Autodesk Fusion 360 part; units mm, degrees
(part 2 of 2)
  line L903 (-140.0079, -18.8092) -> (-138.8476, -19.992)
  line L904 (-137.1524, -16.008) -> (-138.8092, -15.9921)
  line L905 (-138.8092, -15.9921) -> (-139.992, -17.1524)
  line L906 (-139.992, -17.1524) -> (-140.0079, -18.8092)
  line L907 (-137.1908, -20.0079) -> (-136.008, -18.8476)
  line L908 (-146.8476, -19.992) -> (-145.1908, -20.0079)
  line L909 (-144.008, -18.8476) -> (-143.9921, -17.1908)
  line L910 (-143.9921, -17.1908) -> (-145.1524, -16.008)
  line L911 (-148.0079, -18.8092) -> (-146.8476, -19.992)
  line L912 (-145.1524, -16.008) -> (-146.8092, -15.9921)
  line L913 (-146.8092, -15.9921) -> (-147.992, -17.1524)
  line L914 (-147.992, -17.1524) -> (-148.0079, -18.8092)
  line L915 (-145.1908, -20.0079) -> (-144.008, -18.8476)
  line L916 (-154.8476, -19.992) -> (-153.1908, -20.0079)
  line L917 (-152.008, -18.8476) -> (-151.9921, -17.1908)
  line L918 (-151.9921, -17.1908) -> (-153.1524, -16.008)
  line L919 (-156.0079, -18.8092) -> (-154.8476, -19.992)
  line L920 (-153.1524, -16.008) -> (-154.8092, -15.9921)
  line L921 (-154.8092, -15.9921) -> (-155.992, -17.1524)
  line L922 (-155.992, -17.1524) -> (-156.0079, -18.8092)
  line L923 (-153.1908, -20.0079) -> (-152.008, -18.8476)
  line L924 (-162.8476, -19.992) -> (-161.1908, -20.0079)
  line L925 (-160.008, -18.8476) -> (-159.9921, -17.1908)
  line L926 (-159.9921, -17.1908) -> (-161.1524, -16.008)
  line L927 (-164.0079, -18.8092) -> (-162.8476, -19.992)
  line L928 (-161.1524, -16.008) -> (-162.8092, -15.9921)
  line L929 (-162.8092, -15.9921) -> (-163.992, -17.1524)
  line L930 (-163.992, -17.1524) -> (-164.0079, -18.8092)
  line L931 (-161.1908, -20.0079) -> (-160.008, -18.8476)
  line L932 (-170.8476, -19.992) -> (-169.1908, -20.0079)
  line L933 (-168.008, -18.8476) -> (-167.9921, -17.1908)
  line L934 (-167.9921, -17.1908) -> (-169.1524, -16.008)
  line L935 (-172.0079, -18.8092) -> (-170.8476, -19.992)
  line L936 (-169.1524, -16.008) -> (-170.8092, -15.9921)
  line L937 (-170.8092, -15.9921) -> (-171.992, -17.1524)
  line L938 (-171.992, -17.1524) -> (-172.0079, -18.8092)
  line L939 (-169.1908, -20.0079) -> (-168.008, -18.8476)
  line L940 (-10.8476, -11.992) -> (-9.1908, -12.0079)
  line L941 (-8.008, -10.8476) -> (-7.9921, -9.1908)
  line L942 (-7.9921, -9.1908) -> (-9.1524, -8.008)
  line L943 (-12.0079, -10.8092) -> (-10.8476, -11.992)
  line L944 (-9.1524, -8.008) -> (-10.8092, -7.9921)
  line L945 (-10.8092, -7.9921) -> (-11.992, -9.1524)
  line L946 (-11.992, -9.1524) -> (-12.0079, -10.8092)
  line L947 (-9.1908, -12.0079) -> (-8.008, -10.8476)
  line L948 (-18.8476, -11.992) -> (-17.1908, -12.0079)
  line L949 (-16.008, -10.8476) -> (-15.9921, -9.1908)
  line L950 (-15.9921, -9.1908) -> (-17.1524, -8.008)
  line L951 (-20.0079, -10.8092) -> (-18.8476, -11.992)
  line L952 (-17.1524, -8.008) -> (-18.8092, -7.9921)
  line L953 (-18.8092, -7.9921) -> (-19.992, -9.1524)
  line L954 (-19.992, -9.1524) -> (-20.0079, -10.8092)
  line L955 (-17.1908, -12.0079) -> (-16.008, -10.8476)
  line L956 (-26.8476, -11.992) -> (-25.1908, -12.0079)
  line L957 (-24.008, -10.8476) -> (-23.9921, -9.1908)
  line L958 (-23.9921, -9.1908) -> (-25.1524, -8.008)
  line L959 (-28.0079, -10.8092) -> (-26.8476, -11.992)
  line L960 (-25.1524, -8.008) -> (-26.8092, -7.9921)
  line L961 (-26.8092, -7.9921) -> (-27.992, -9.1524)
  line L962 (-27.992, -9.1524) -> (-28.0079, -10.8092)
  line L963 (-25.1908, -12.0079) -> (-24.008, -10.8476)
  line L964 (-34.8476, -11.992) -> (-33.1908, -12.0079)
  line L965 (-32.008, -10.8476) -> (-31.9921, -9.1908)
  line L966 (-31.9921, -9.1908) -> (-33.1524, -8.008)
  line L967 (-36.0079, -10.8092) -> (-34.8476, -11.992)
  line L968 (-33.1524, -8.008) -> (-34.8092, -7.9921)
  line L969 (-34.8092, -7.9921) -> (-35.992, -9.1524)
  line L970 (-35.992, -9.1524) -> (-36.0079, -10.8092)
  line L971 (-33.1908, -12.0079) -> (-32.008, -10.8476)
  line L972 (-42.8476, -11.992) -> (-41.1908, -12.0079)
  line L973 (-40.008, -10.8476) -> (-39.9921, -9.1908)
  line L974 (-39.9921, -9.1908) -> (-41.1524, -8.008)
  line L975 (-44.0079, -10.8092) -> (-42.8476, -11.992)
  line L976 (-41.1524, -8.008) -> (-42.8092, -7.9921)
  line L977 (-42.8092, -7.9921) -> (-43.992, -9.1524)
  line L978 (-43.992, -9.1524) -> (-44.0079, -10.8092)
  line L979 (-41.1908, -12.0079) -> (-40.008, -10.8476)
  line L980 (-50.8476, -11.992) -> (-49.1908, -12.0079)
  line L981 (-48.008, -10.8476) -> (-47.9921, -9.1908)
  line L982 (-47.9921, -9.1908) -> (-49.1524, -8.008)
  line L983 (-52.0079, -10.8092) -> (-50.8476, -11.992)
  line L984 (-49.1524, -8.008) -> (-50.8092, -7.9921)
  line L985 (-50.8092, -7.9921) -> (-51.992, -9.1524)
  line L986 (-51.992, -9.1524) -> (-52.0079, -10.8092)
  line L987 (-49.1908, -12.0079) -> (-48.008, -10.8476)
  line L988 (-58.8476, -11.992) -> (-57.1908, -12.0079)
  line L989 (-56.008, -10.8476) -> (-55.9921, -9.1908)
  line L990 (-55.9921, -9.1908) -> (-57.1524, -8.008)
  line L991 (-60.0079, -10.8092) -> (-58.8476, -11.992)
  line L992 (-57.1524, -8.008) -> (-58.8092, -7.9921)
  line L993 (-58.8092, -7.9921) -> (-59.992, -9.1524)
  line L994 (-59.992, -9.1524) -> (-60.0079, -10.8092)
  line L995 (-57.1908, -12.0079) -> (-56.008, -10.8476)
  line L996 (-66.8476, -11.992) -> (-65.1908, -12.0079)
  line L997 (-64.008, -10.8476) -> (-63.9921, -9.1908)
  line L998 (-63.9921, -9.1908) -> (-65.1524, -8.008)
  line L999 (-68.0079, -10.8092) -> (-66.8476, -11.992)
  line L1000 (-65.1524, -8.008) -> (-66.8092, -7.9921)
  line L1001 (-66.8092, -7.9921) -> (-67.992, -9.1524)
  line L1002 (-67.992, -9.1524) -> (-68.0079, -10.8092)
  line L1003 (-65.1908, -12.0079) -> (-64.008, -10.8476)
  line L1004 (-74.8476, -11.992) -> (-73.1908, -12.0079)
  line L1005 (-72.008, -10.8476) -> (-71.9921, -9.1908)
  line L1006 (-71.9921, -9.1908) -> (-73.1524, -8.008)
  line L1007 (-76.0079, -10.8092) -> (-74.8476, -11.992)
  line L1008 (-73.1524, -8.008) -> (-74.8092, -7.9921)
  line L1009 (-74.8092, -7.9921) -> (-75.992, -9.1524)
  line L1010 (-75.992, -9.1524) -> (-76.0079, -10.8092)
  line L1011 (-73.1908, -12.0079) -> (-72.008, -10.8476)
  line L1012 (-82.8476, -11.992) -> (-81.1908, -12.0079)
  line L1013 (-80.008, -10.8476) -> (-79.9921, -9.1908)
  line L1014 (-79.9921, -9.1908) -> (-81.1524, -8.008)
  line L1015 (-84.0079, -10.8092) -> (-82.8476, -11.992)
  line L1016 (-81.1524, -8.008) -> (-82.8092, -7.9921)
  line L1017 (-82.8092, -7.9921) -> (-83.992, -9.1524)
  line L1018 (-83.992, -9.1524) -> (-84.0079, -10.8092)
  line L1019 (-81.1908, -12.0079) -> (-80.008, -10.8476)
  line L1020 (-90.8476, -11.992) -> (-89.1908, -12.0079)
  line L1021 (-88.008, -10.8476) -> (-87.9921, -9.1908)
  line L1022 (-87.9921, -9.1908) -> (-89.1524, -8.008)
  line L1023 (-92.0079, -10.8092) -> (-90.8476, -11.992)
  line L1024 (-89.1524, -8.008) -> (-90.8092, -7.9921)
  line L1025 (-90.8092, -7.9921) -> (-91.992, -9.1524)
  line L1026 (-91.992, -9.1524) -> (-92.0079, -10.8092)
  line L1027 (-89.1908, -12.0079) -> (-88.008, -10.8476)
  line L1028 (-98.8476, -11.992) -> (-97.1908, -12.0079)
  line L1029 (-96.008, -10.8476) -> (-95.9921, -9.1908)
  line L1030 (-95.9921, -9.1908) -> (-97.1524, -8.008)
  line L1031 (-100.0079, -10.8092) -> (-98.8476, -11.992)
  line L1032 (-97.1524, -8.008) -> (-98.8092, -7.9921)
  line L1033 (-98.8092, -7.9921) -> (-99.992, -9.1524)
  line L1034 (-99.992, -9.1524) -> (-100.0079, -10.8092)
  line L1035 (-97.1908, -12.0079) -> (-96.008, -10.8476)
  line L1036 (-106.8476, -11.992) -> (-105.1908, -12.0079)
  line L1037 (-104.008, -10.8476) -> (-103.9921, -9.1908)
  line L1038 (-103.9921, -9.1908) -> (-105.1524, -8.008)
  line L1039 (-108.0079, -10.8092) -> (-106.8476, -11.992)
  line L1040 (-105.1524, -8.008) -> (-106.8092, -7.9921)
  line L1041 (-106.8092, -7.9921) -> (-107.992, -9.1524)
  line L1042 (-107.992, -9.1524) -> (-108.0079, -10.8092)
  line L1043 (-105.1908, -12.0079) -> (-104.008, -10.8476)
  line L1044 (-114.8476, -11.992) -> (-113.1908, -12.0079)
  line L1045 (-112.008, -10.8476) -> (-111.9921, -9.1908)
  line L1046 (-111.9921, -9.1908) -> (-113.1524, -8.008)
  line L1047 (-116.0079, -10.8092) -> (-114.8476, -11.992)
  line L1048 (-113.1524, -8.008) -> (-114.8092, -7.9921)
  line L1049 (-114.8092, -7.9921) -> (-115.992, -9.1524)
  line L1050 (-115.992, -9.1524) -> (-116.0079, -10.8092)
  line L1051 (-113.1908, -12.0079) -> (-112.008, -10.8476)
  line L1052 (-122.8476, -11.992) -> (-121.1908, -12.0079)
  line L1053 (-120.008, -10.8476) -> (-119.9921, -9.1908)
  line L1054 (-119.9921, -9.1908) -> (-121.1524, -8.008)
  line L1055 (-124.0079, -10.8092) -> (-122.8476, -11.992)
  line L1056 (-121.1524, -8.008) -> (-122.8092, -7.9921)
  line L1057 (-122.8092, -7.9921) -> (-123.992, -9.1524)
  line L1058 (-123.992, -9.1524) -> (-124.0079, -10.8092)
  line L1059 (-121.1908, -12.0079) -> (-120.008, -10.8476)
  line L1060 (-130.8476, -11.992) -> (-129.1908, -12.0079)
  line L1061 (-128.008, -10.8476) -> (-127.9921, -9.1908)
  line L1062 (-127.9921, -9.1908) -> (-129.1524, -8.008)
  line L1063 (-132.0079, -10.8092) -> (-130.8476, -11.992)
  line L1064 (-129.1524, -8.008) -> (-130.8092, -7.9921)
  line L1065 (-130.8092, -7.9921) -> (-131.992, -9.1524)
  line L1066 (-131.992, -9.1524) -> (-132.0079, -10.8092)
  line L1067 (-129.1908, -12.0079) -> (-128.008, -10.8476)
  line L1068 (-138.8476, -11.992) -> (-137.1908, -12.0079)
  line L1069 (-136.008, -10.8476) -> (-135.9921, -9.1908)
  line L1070 (-135.9921, -9.1908) -> (-137.1524, -8.008)
  line L1071 (-140.0079, -10.8092) -> (-138.8476, -11.992)
  line L1072 (-137.1524, -8.008) -> (-138.8092, -7.9921)
  line L1073 (-138.8092, -7.9921) -> (-139.992, -9.1524)
  line L1074 (-139.992, -9.1524) -> (-140.0079, -10.8092)
  line L1075 (-137.1908, -12.0079) -> (-136.008, -10.8476)
  line L1076 (-146.8476, -11.992) -> (-145.1908, -12.0079)
  line L1077 (-144.008, -10.8476) -> (-143.9921, -9.1908)
  line L1078 (-143.9921, -9.1908) -> (-145.1524, -8.008)
  line L1079 (-148.0079, -10.8092) -> (-146.8476, -11.992)
  line L1080 (-145.1524, -8.008) -> (-146.8092, -7.9921)
  line L1081 (-146.8092, -7.9921) -> (-147.992, -9.1524)
  line L1082 (-147.992, -9.1524) -> (-148.0079, -10.8092)
  line L1083 (-145.1908, -12.0079) -> (-144.008, -10.8476)
  line L1084 (-154.8476, -11.992) -> (-153.1908, -12.0079)
  line L1085 (-152.008, -10.8476) -> (-151.9921, -9.1908)
  line L1086 (-151.9921, -9.1908) -> (-153.1524, -8.008)
  line L1087 (-156.0079, -10.8092) -> (-154.8476, -11.992)
  line L1088 (-153.1524, -8.008) -> (-154.8092, -7.9921)
  line L1089 (-154.8092, -7.9921) -> (-155.992, -9.1524)
  line L1090 (-155.992, -9.1524) -> (-156.0079, -10.8092)
  line L1091 (-153.1908, -12.0079) -> (-152.008, -10.8476)
  line L1092 (-162.8476, -11.992) -> (-161.1908, -12.0079)
  line L1093 (-160.008, -10.8476) -> (-159.9921, -9.1908)
  line L1094 (-159.9921, -9.1908) -> (-161.1524, -8.008)
  line L1095 (-164.0079, -10.8092) -> (-162.8476, -11.992)
  line L1096 (-161.1524, -8.008) -> (-162.8092, -7.9921)
  line L1097 (-162.8092, -7.9921) -> (-163.992, -9.1524)
  line L1098 (-163.992, -9.1524) -> (-164.0079, -10.8092)
  line L1099 (-161.1908, -12.0079) -> (-160.008, -10.8476)
  line L1100 (-170.8476, -11.992) -> (-169.1908, -12.0079)
  line L1101 (-168.008, -10.8476) -> (-167.9921, -9.1908)
  line L1102 (-167.9921, -9.1908) -> (-169.1524, -8.008)
  line L1103 (-172.0079, -10.8092) -> (-170.8476, -11.992)
  line L1104 (-169.1524, -8.008) -> (-170.8092, -7.9921)
  line L1105 (-170.8092, -7.9921) -> (-171.992, -9.1524)
  line L1106 (-171.992, -9.1524) -> (-172.0079, -10.8092)
  line L1107 (-169.1908, -12.0079) -> (-168.008, -10.8476)
  point P0 (-10, -50)
  point P1 (-18, -50)
  point P2 (-26, -50)
  point P3 (-34, -50)
  point P4 (-42, -50)
  point P5 (-50, -50)
  point P6 (-58, -50)
  point P7 (-66, -50)
  point P8 (-74, -50)
  point P9 (-82, -50)
  point P10 (-90, -50)
  point P11 (-98, -50)
  point P12 (-106, -50)
  point P13 (-114, -50)
  point P14 (-122, -50)
  point P15 (-130, -50)
  point P16 (-138, -50)
  point P17 (-146, -50)
  point P18 (-154, -50)
  point P19 (-162, -50)
  point P20 (-170, -50)
  point P21 (-10, -42)
  point P22 (-18, -42)
  point P23 (-26, -42)
  point P24 (-34, -42)
  point P25 (-42, -42)
  point P26 (-50, -42)
  point P27 (-58, -42)
  point P28 (-66, -42)
  point P29 (-74, -42)
  point P30 (-82, -42)
  point P31 (-90, -42)
  point P32 (-98, -42)
  point P33 (-106, -42)
  point P34 (-114, -42)
  point P35 (-122, -42)
  point P36 (-130, -42)
  point P37 (-138, -42)
  point P38 (-146, -42)
  point P39 (-154, -42)
  point P40 (-162, -42)
  point P41 (-170, -42)
  point P42 (-10, -34)
  point P43 (-18, -34)
  point P44 (-26, -34)
  point P45 (-34, -34)
  point P46 (-42, -34)
  point P47 (-50, -34)
  point P48 (-58, -34)
  point P49 (-66, -34)
  point P50 (-74, -34)
  point P51 (-82, -34)
  point P52 (-90, -34)
  point P53 (-98, -34)
  point P54 (-106, -34)
  point P55 (-114, -34)
  point P56 (-122, -34)
  point P57 (-130, -34)
  point P58 (-138, -34)
  point P59 (-146, -34)
  point P60 (-154, -34)
  point P61 (-162, -34)
  point P62 (-170, -34)
  point P63 (-10, -26)
  point P64 (-18, -26)
  point P65 (-26, -26)
  point P66 (-34, -26)
  point P67 (-42, -26)
  point P68 (-50, -26)
  point P69 (-58, -26)
  point P70 (-66, -26)
  point P71 (-74, -26)
  point P72 (-82, -26)
  point P73 (-90, -26)
  point P74 (-98, -26)
  point P75 (-106, -26)
  point P76 (-114, -26)
  point P77 (-122, -26)
  point P78 (-130, -26)
  point P79 (-138, -26)
  point P80 (-146, -26)
  point P81 (-154, -26)
  point P82 (-162, -26)
  point P83 (-170, -26)
  point P84 (-10, -18)
  point P85 (-18, -18)
  point P86 (-26, -18)
  point P87 (-34, -18)
  point P88 (-42, -18)
  point P89 (-50, -18)
  point P90 (-58, -18)
  point P91 (-66, -18)
  point P92 (-74, -18)
  point P93 (-82, -18)
  point P94 (-90, -18)
  point P95 (-98, -18)
  point P96 (-106, -18)
  point P97 (-114, -18)
  point P98 (-122, -18)
  point P99 (-130, -18)
  point P100 (-138, -18)
  point P101 (-146, -18)
  point P102 (-154, -18)
  point P103 (-162, -18)
  point P104 (-170, -18)
  point P105 (-10, -10)
  point P106 (-18, -10)
  point P107 (-26, -10)
  point P108 (-34, -10)
  point P109 (-42, -10)
  point P110 (-50, -10)
  point P111 (-58, -10)
  point P112 (-66, -10)
  point P113 (-74, -10)
  point P114 (-82, -10)
  point P115 (-90, -10)
  point P116 (-98, -10)
  point P117 (-106, -10)
  point P118 (-114, -10)
  point P119 (-122, -10)
  point P120 (-130, -10)
  point P121 (-138, -10)
  point P122 (-146, -10)
  point P123 (-154, -10)
  point P124 (-162, -10)
  point P125 (-170, -10)
  dimension "d5" = 5
  dimension "d6" = 2
  dimension "d9" = -20
  dimension "d10" = -54
  dimension "d11" = 5
  dimension "d12" = 2
  dimension "d13" = 2
  dimension "d14" = 2
  dimension "d15" = 10
  dimension "d18" = -174
  dimension "d19" = -20
  dimension "d39" = 2
  dimension "d40" = 10
  dimension "d41" = 10
  dimension "d44" = -8
  dimension "d45" = 8
  constraint horizontal L4
  constraint vertical L5
  constraint horizontal L6
  constraint vertical L7
  constraint horizontal L76
  constraint vertical L77
  constraint horizontal L78
  constraint vertical L79
  measures "d5" distance of L0 L7
  measures "d6" distance of L1 L4
  measures "d11" distance of L1 L76
  measures "d12" distance of L0 L79
  measures "d13" distance of L76.start L76.end
  measures "d14" distance of L4.start L6.end
  measures "d15" distance of L76.start L78.end
  measures "d39" distance of P0 L107
  measures "d40" distance of L3 P0
  measures "d41" distance of L0 P0
extrude "Extrude2" cut sketch "Sketch2" against normal blind 5 contours L4 L5 L6 L7 | L8 L9 L10 L11 | L12 L13 L14 L15 | L16 L17 L18 L19 | L20 L21 L22 L23 | L24 L25 L26 L27 | L28 L29 L30 L31 | L32 L33 L34 L35 | L36 L37 L38 L39 | L40 L41 L42 L43 | L44 L45 L46 L47 | L48 L49 L50 L51 | L52 L53 L54 L55 | L56 L57 L58 L59 | L60 L61 L62 L63 | L64 L65 L66 L67 | L68 L69 L70 L71 | L72 L73 L74 L75 | L76 L77 L78 L79 | L80 L81 L82 L83 | L84 L85 L86 L87 | L88 L89 L90 L91 | L92 L93 L94 L95 | L96 L97 L98 L99 | L100 L101 L102 L103 L104 L105 L106 L107 | L108 L109 L110 L111 L112 L113 L114 L115 | L116 L117 L118 L119 L120 L121 L122 L123 | L124 L125 L126 L127 L128 L129 L130 L131 | L132 L133 L134 L135 L136 L137 L138 L139 | L140 L141 L142 L143 L144 L145 L146 L147 | L148 L149 L150 L151 L152 L153 L154 L155 | L156 L157 L158 L159 L160 L161 L162 L163 | L164 L165 L166 L167 L168 L169 L170 L171 | L172 L173 L174 L175 L176 L177 L178 L179 | L180 L181 L182 L183 L184 L185 L186 L187 | L188 L189 L190 L191 L192 L193 L194 L195 | L196 L197 L198 L199 L200 L201 L202 L203 | L204 L205 L206 L207 L208 L209 L210 L211 | L212 L213 L214 L215 L216 L217 L218 L219 | L220 L221 L222 L223 L224 L225 L226 L227 | L228 L229 L230 L231 L232 L233 L234 L235 | L236 L237 L238 L239 L240 L241 L242 L243 | L244 L245 L246 L247 L248 L249 L250 L251 | L252 L253 L254 L255 L256 L257 L258 L259 | L260 L261 L262 L263 L264 L265 L266 L267 | L268 L269 L270 L271 L272 L273 L274 L275 | L276 L277 L278 L279 L280 L281 L282 L283 | L284 L285 L286 L287 L288 L289 L290 L291 | L292 L293 L294 L295 L296 L297 L298 L299 | L300 L301 L302 L303 L304 L305 L306 L307 | L308 L309 L310 L311 L312 L313 L314 L315 | L316 L317 L318 L319 L320 L321 L322 L323 | L324 L325 L326 L327 L328 L329 L330 L331 | L332 L333 L334 L335 L336 L337 L338 L339 | L340 L341 L342 L343 L344 L345 L346 L347 | L348 L349 L350 L351 L352 L353 L354 L355 | L356 L357 L358 L359 L360 L361 L362 L363 | L364 L365 L366 L367 L368 L369 L370 L371 | L372 L373 L374 L375 L376 L377 L378 L379 | L380 L381 L382 L383 L384 L385 L386 L387 | L388 L389 L390 L391 L392 L393 L394 L395 | L396 L397 L398 L399 L400 L401 L402 L403 | L404 L405 L406 L407 L408 L409 L410 L411 | L412 L413 L414 L415 L416 L417 L418 L419 | L420 L421 L422 L423 L424 L425 L426 L427 | L428 L429 L430 L431 L432 L433 L434 L435 | L436 L437 L438 L439 L440 L441 L442 L443 | L444 L445 L446 L447 L448 L449 L450 L451 | L452 L453 L454 L455 L456 L457 L458 L459 | L460 L461 L462 L463 L464 L465 L466 L467 | L468 L469 L470 L471 L472 L473 L474 L475 | L476 L477 L478 L479 L480 L481 L482 L483 | L484 L485 L486 L487 L488 L489 L490 L491 | L492 L493 L494 L495 L496 L497 L498 L499 | L500 L501 L502 L503 L504 L505 L506 L507 | L508 L509 L510 L511 L512 L513 L514 L515 | L516 L517 L518 L519 L520 L521 L522 L523 | L524 L525 L526 L527 L528 L529 L530 L531 | L532 L533 L534 L535 L536 L537 L538 L539 | L540 L541 L542 L543 L544 L545 L546 L547 | L548 L549 L550 L551 L552 L553 L554 L555 | L556 L557 L558 L559 L560 L561 L562 L563 | L564 L565 L566 L567 L568 L569 L570 L571 | L572 L573 L574 L575 L576 L577 L578 L579 | L580 L581 L582 L583 L584 L585 L586 L587 | L588 L589 L590 L591 L592 L593 L594 L595 | L596 L597 L598 L599 L600 L601 L602 L603 | L604 L605 L606 L607 L608 L609 L610 L611 | L612 L613 L614 L615 L616 L617 L618 L619 | L620 L621 L622 L623 L624 L625 L626 L627 | L628 L629 L630 L631 L632 L633 L634 L635 | L636 L637 L638 L639 L640 L641 L642 L643 | L644 L645 L646 L647 L648 L649 L650 L651 | L652 L653 L654 L655 L656 L657 L658 L659 | L660 L661 L662 L663 L664 L665 L666 L667 | L668 L669 L670 L671 L672 L673 L674 L675 | L676 L677 L678 L679 L680 L681 L682 L683 | L684 L685 L686 L687 L688 L689 L690 L691 | L692 L693 L694 L695 L696 L697 L698 L699 | L700 L701 L702 L703 L704 L705 L706 L707 | L708 L709 L710 L711 L712 L713 L714 L715 | L716 L717 L718 L719 L720 L721 L722 L723 | L724 L725 L726 L727 L728 L729 L730 L731 | L732 L733 L734 L735 L736 L737 L738 L739 | L740 L741 L742 L743 L744 L745 L746 L747 | L748 L749 L750 L751 L752 L753 L754 L755 | L756 L757 L758 L759 L760 L761 L762 L763 | L764 L765 L766 L767 L768 L769 L770 L771 | L772 L773 L774 L775 L776 L777 L778 L779 | L780 L781 L782 L783 L784 L785 L786 L787 | L788 L789 L790 L791 L792 L793 L794 L795 | L796 L797 L798 L799 L800 L801 L802 L803 | L804 L805 L806 L807 L808 L809 L810 L811 | L812 L813 L814 L815 L816 L817 L818 L819 | L820 L821 L822 L823 L824 L825 L826 L827 | L828 L829 L830 L831 L832 L833 L834 L835 | L836 L837 L838 L839 L840 L841 L842 L843 | L844 L845 L846 L847 L848 L849 L850 L851 | L852 L853 L854 L855 L856 L857 L858 L859 | L860 L861 L862 L863 L864 L865 L866 L867 | L868 L869 L870 L871 L872 L873 L874 L875 | L876 L877 L878 L879 L880 L881 L882 L883 | L884 L885 L886 L887 L888 L889 L890 L891 | L892 L893 L894 L895 L896 L897 L898 L899 | L900 L901 L902 L903 L904 L905 L906 L907 | L908 L909 L910 L911 L912 L913 L914 L915 | L916 L917 L918 L919 L920 L921 L922 L923 | L924 L925 L926 L927 L928 L929 L930 L931 | L932 L933 L934 L935 L936 L937 L938 L939 | L940 L941 L942 L943 L944 L945 L946 L947 | L948 L949 L950 L951 L952 L953 L954 L955 | L956 L957 L958 L959 L960 L961 L962 L963 | L964 L965 L966 L967 L968 L969 L970 L971 | L972 L973 L974 L975 L976 L977 L978 L979 | L980 L981 L982 L983 L984 L985 L986 L987 | L988 L989 L990 L991 L992 L993 L994 L995 | L996 L997 L998 L999 L1000 L1001 L1002 L1003 | L1004 L1005 L1006 L1007 L1008 L1009 L1010 L1011 | L1012 L1013 L1014 L1015 L1016 L1017 L1018 L1019 | L1020 L1021 L1022 L1023 L1024 L1025 L1026 L1027 | L1028 L1029 L1030 L1031 L1032 L1033 L1034 L1035 | L1036 L1037 L1038 L1039 L1040 L1041 L1042 L1043 | L1044 L1045 L1046 L1047 L1048 L1049 L1050 L1051 | L1052 L1053 L1054 L1055 L1056 L1057 L1058 L1059 | L1060 L1061 L1062 L1063 L1064 L1065 L1066 L1067 | L1068 L1069 L1070 L1071 L1072 L1073 L1074 L1075 | L1076 L1077 L1078 L1079 L1080 L1081 L1082 L1083 | L1084 L1085 L1086 L1087 L1088 L1089 L1090 L1091 | L1092 L1093 L1094 L1095 L1096 L1097 L1098 L1099 | L1100 L1101 L1102 L1103 L1104 L1105 L1106 L1107
